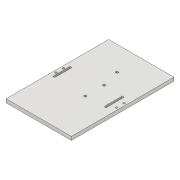
# Autodesk Inventor part: mesa
Saved by Autodesk Inventor 2022 (Build 260153000, 153)
## iProperties
Created: 2018-06-05
Part Number: mesa
Material: MDF Tablero de fibras de densidad media
Document SubType Name: Modeling
Designer: Cristiano
Density: 0.8 g/cm^3
Appearance: Suave - Blanco
Author: Cristiano
Autodesk Inventor part; units mm, degrees
ref_plane "YZ Plane" through (0, 0, 0) normal (1, 0, 0) x (0, 1, 0)
ref_plane "XZ Plane" through (0, 0, 0) normal (0, 1, 0) x (-1, 0, 0)
ref_plane "XY Plane" through (0, 0, 0) normal (0, 0, 1) x (1, 0, 0)
sketch "Boceto1" plane through (0, 0, 0) normal (0, 1, 0) x (-1, 0, 0)
  line L0 (0, 0) -> (550, 0)
  line L1 (550, 0) -> (550, -350)
  line L2 (550, -350) -> (0, -350)
  line L3 (0, -350) -> (0, 0)
  line L4 (0, -175) -> (550, -175) construction
  line L5 (275, -350) -> (275, 0) construction
  circle A0 centre (255, -12.5) radius 5
  circle A1 centre (295, -12.5) radius 5
  circle A2 centre (255, -337.5) radius 5
  circle A3 centre (295, -337.5) radius 5
  dimension "d0" = 350
  dimension "d1" = 550
  dimension "d83" = 12.5
  dimension "d84" = 10
  dimension "d85" = 20
  dimension "d88" = 40
  dimension "d95" = 325
  constraints: 12 end point, 4 centre point, 4 midpoint, 2 horizontal, 2 parallel, 1 perpendicular, 1 vertical, 6 other
  measures "d0" distance of L2.end L0.start
  measures "d1" distance of L0.start L0.end
  measures "d83" distance from line of L0 A0.centre
  measures "d84" diameter of A0
  measures "d85" distance from line of L5 A0.centre
  measures "d88" distance of A0.centre A1.centre
  measures "d95" distance of A0.centre A2.centre
extrude "Extrusión10" add sketch "Boceto1" along normal blind 19
sketch "Boceto8" plane through (0, 19, 0) normal (0, 1, 0) x (1, 0, 0)
  line L0 (-550, 0) -> (0, 0) construction
  line L1 (-275, 0) -> (-275, 350) construction
  line L2 (0, 350) -> (-550, 350) construction
  circle A0 centre (-224.5, 200) radius 6.5
  circle A1 centre (-325.5, 200) radius 6.5
  dimension "d102" = 101
  dimension "d103" = 50.5
  dimension "d104" = 13
  dimension "d116" = 150
  constraints: 2 centre point, 2 end point, 2 midpoint, 1 equal radius, 1 horizontal alignment
  measures "d102" distance of A1.centre A0.centre
  measures "d103" distance from line of L1 A1.centre
  measures "d104" diameter of A0
  measures "d116" distance from line of L2 A0.centre
extrude "Extrusión11" cut sketch "Boceto8" against normal through all
sketch "Boceto9" plane through (0, 0, 0) normal (0, -1, 0) x (1, 0, 0)
  line L0 (0, -305) -> (-550, -305) construction
  line L1 (-550, -350) -> (-550, 0) construction
  line L2 (0, -350) -> (-550, -350) construction
  line L3 (-230, -305) -> (-320, -305) construction
  line L4 (-230, -300) -> (-320, -300)
  line L5 (-320, -310) -> (-230, -310)
  arc A0 (-230, -310) -> (-230, -300) centre (-230, -305) ccw
  arc A1 (-320, -300) -> (-320, -310) centre (-320, -305) ccw
  line L6 (0, 0) -> (0, -350) construction
  line L7 (0, 0) -> (0, -350) projected
  line L8 (0, -27) -> (-550, -27) construction
  line L9 (-550, 0) -> (0, 0) projected
  line L10 (-232.5, -27) -> (-317.5, -27) construction
  line L11 (-232.5, -22) -> (-317.5, -22)
  line L12 (-317.5, -32) -> (-232.5, -32)
  arc A2 (-232.5, -32) -> (-232.5, -22) centre (-232.5, -27) ccw
  arc A3 (-317.5, -22) -> (-317.5, -32) centre (-317.5, -27) ccw
  point P0 (-275, -305)
  point P1 (-275, -305)
  point P2 (-275, -27)
  point P3 (-275, -27)
  dimension "d108" = 45
  dimension "d109" = 10
  dimension "d110" = 90
  dimension "d111" = 27
  dimension "d112" = 10
  dimension "d113" = 85
  constraints: 20 end point, 8 point on circle, 8 point on line, 8 tangent, 4 centre point, 4 midpoint, 2 coincident, 2 parallel, 1 horizontal, 1 perpendicular
  measures "d108" distance between parallel lines of L2 L0
  measures "d109" distance between parallel lines of L4 L5
  measures "d110" distance of L3.end L3.start
  measures "d111" distance between parallel lines of L9 L8
  measures "d112" distance between parallel lines of L11 L12
  measures "d113" distance of L10.end L10.start
extrude "Extrusión12" cut sketch "Boceto9" against normal through all
sketch "Sketch10" plane through (0, 0, 0) normal (0, -1, 0) x (1, 0, 0)
  line L0 (-135, -169) -> (-125, -169)
  line L1 (-125, -169) -> (-125, -181)
  line L2 (-125, -181) -> (-135, -181)
  line L3 (-135, -181) -> (-135, -169)
  circle A0 centre (-295, -337.5) radius 5 projected
  line L4 (-550, -350) -> (-550, 0) projected
  circle A1 centre (-255, -337.5) radius 5 projected
  point P0 (0, 0)
  point P1 (-135, -175)
  point P2 (-550, -175)
  dimension "d117" = 10
  dimension "d118" = 12
  dimension "d122" = 120
  constraints: 8 end point, 2 midpoint, 2 parallel, 1 horizontal, 1 horizontal alignment, 1 perpendicular
  measures "d117" distance of L1.end L2.end
  measures "d118" distance of L0.end L1.end
  measures "d122" horizontal distance of L2.end A1.centre
extrude "Extrusion13" cut sketch "Sketch10" against normal through all contours L0 L1 L2 L3
